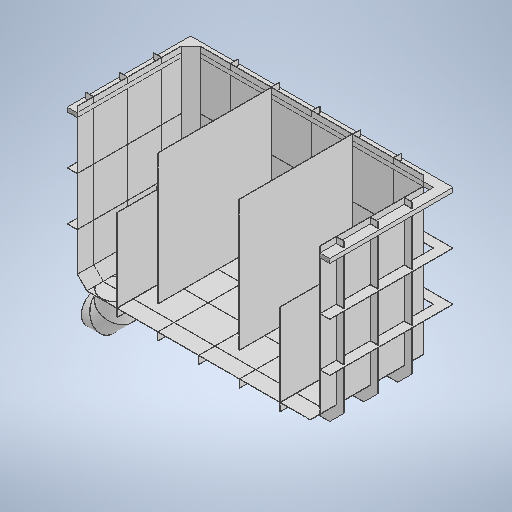
# Autodesk Inventor part: GBK-RK-0003 RK dummy 3
Saved by Autodesk Inventor 2026.2 (Build 302298000, 298)
## iProperties
Created: 2026-08-26
Part Number: GBK-RK-0003 RK dummy 3
Material: Stainless Steel
Document SubType Name: Modeling
Designer: admin
Density: 8 g/cm^3
Appearance: Default
Author: admin
Autodesk Inventor part; units mm, degrees
ref_plane "YZ Plane" through (0, 0, 0) normal (1, 0, 0) x (0, 1, 0)
ref_plane "XZ Plane" through (0, 0, 0) normal (0, 1, 0) x (-1, 0, 0)
ref_plane "XY Plane" through (0, 0, 0) normal (0, 0, 1) x (1, 0, 0)
sketch "Sketch1" plane through (0, 0, 0) normal (0, 1, 0) x (-1, 0, 0)
  line L0 (1250, 650) -> (-1250, 650)
  line L1 (-1250, 650) -> (-1250, -650)
  line L2 (-1250, -650) -> (1250, -650)
  line L3 (1250, -650) -> (1250, 650)
  line L4 (1250, 650) -> (-1250, -650) construction
  line L5 (-1250, 650) -> (1250, -650) construction
  point P0 (0, 0)
  dimension "d0" = 2500
  dimension "d1" = 1300
  constraints: 12 end point, 2 midpoint, 2 parallel, 1 horizontal, 1 perpendicular
  measures "d0" distance of L2.end L1.end
  measures "d1" distance of L1.end L0.end
extrude "Extrusion1" add sketch "Sketch1" along normal blind 100 and the other way blind 1500
chamfer "Chamfer1" distance 100 angle 45 8 edges at (0, -1500, 650) (1250, -1500, 0) (0, -1500, -650) (-1250, -1500, 0) (-1250, -700, 650) (-1250, -700, -650) (1250, -700, -650) (1250, -700, 650)
shell "Shell1" thickness 4 removed faces 1 at (383.3333, 100, -216.6667)
sketch "Sketch4" plane through (0, 0, 0) normal (0, 0, 1) x (1, 0, 0)
  line L0 (-1250, -1400) -> (-1250, 100) projected
  line L1 (-1250, 100) -> (-1250, -1400) projected
  line L2 (-1250, -1400) -> (-1150, -1500) projected
  line L3 (-1150, -1500) -> (-1250, -1400) projected
  line L4 (1150, -1500) -> (-1150, -1500) projected
  line L5 (-1150, -1500) -> (1150, -1500) projected
  line L6 (1250, -1400) -> (1150, -1500) projected
  line L7 (1150, -1500) -> (1250, -1400) projected
  line L8 (1250, 100) -> (1250, -1400) projected
  line L9 (1250, -1400) -> (1250, 100) projected
  line L10 (-1250, 100) -> (-1330, 100)
  line L11 (-1330, 100) -> (-1330, -1433.1371)
  line L12 (-1330, -1433.1371) -> (-1183.1371, -1580)
  line L13 (-1183.1371, -1580) -> (1183.1371, -1580)
  line L14 (1183.1371, -1580) -> (1330, -1433.1371)
  line L15 (1330, -1433.1371) -> (1330, 100)
  line L16 (1330, 100) -> (1250, 100)
  line L17 (0, -1500) -> (0, -1580) construction
  line L18 (-1200, -1450) -> (-1256.5685, -1506.5685) construction
  line L19 (1200, -1450) -> (1256.5685, -1506.5685) construction
  point P0 (0, 0)
  dimension "d16" = 80
  constraints: 20 end point, 7 perpendicular, 6 midpoint, 2 equal length, 2 parallel, 1 point on line
  measures "d16" distance of L1.start L10.end
sketch "Sketch2" plane through (0, 0, 0) normal (1, 0, 0) x (0, 1, 0)
  line L0 (100, -650) -> (100, 650) construction
  line L1 (100, 650) -> (100, 730)
  line L2 (100, 730) -> (-1433.1371, 730)
  line L3 (-1433.1371, 730) -> (-1580, 583.1371)
  line L4 (-1580, 583.1371) -> (-1580, -583.1371)
  line L5 (-1580, -583.1371) -> (-1433.1371, -730)
  line L6 (-1433.1371, -730) -> (100, -730)
  line L7 (100, -730) -> (100, -650)
  line L8 (-1450, -600) -> (-1506.5685, -656.5685) construction
  line L9 (-1500, 0) -> (-1580, 0) construction
  line L10 (-1450, 600) -> (-1506.5685, 656.5685) construction
  line L11 (-1400, -650) -> (-1500, -550)
  line L12 (-1500, -550) -> (-1400, -650) projected
  line L13 (-1400, 650) -> (-1500, 550)
  line L14 (-1500, 550) -> (-1400, 650) projected
  line L15 (-1400, 650) -> (100, 650)
  line L16 (100, 650) -> (-1400, 650) projected
  line L17 (100, -650) -> (-1400, -650)
  line L18 (-1400, -650) -> (100, -650) projected
  line L19 (-1500, -550) -> (-1500, 550) projected
  line L20 (-1500, 550) -> (-1500, -550) projected
  point P0 (0, 0)
  dimension "d10" = 80
  constraints: 30 end point, 6 midpoint, 6 perpendicular, 4 equal length, 2 parallel, 2 point on line
  measures "d10" distance of L0.end L1.end
extrude "Extrusion4" add sketch "Sketch4" along normal mid plane 4
extrude "Extrusion5" add sketch "Sketch2" along normal mid plane 4
pattern_linear "Rectangular Pattern2" count 5 spacing 420 along (1, 0, 0) of "Extrusion5" first direction both ways yes
pattern_linear "Rectangular Pattern3" count 3 spacing 350 along (0, 0, 1) of "Extrusion4" first direction both ways yes
sketch "Sketch5" plane through (0, 0, 0) normal (0, 1, 0) x (-1, 0, 0)
  line L0 (-1246, -548.3431) -> (-1246, 548.3431) projected
  line L1 (-1148.3431, -646) -> (-1246, -548.3431) projected
  line L2 (-1250, -650) -> (1250, -650)
  line L3 (1250, -650) -> (1250, 650)
  line L4 (1250, 650) -> (-1250, 650)
  line L5 (-1250, 650) -> (-1250, -650)
  line L6 (-1250, -650) -> (1250, 650) construction
  line L7 (1250, -650) -> (-1250, 650) construction
  line L8 (1150, 650) -> (842, 650) projected
  line L9 (1250, 352) -> (1250, 550) projected
  line L10 (-1350, -750) -> (1350, -750)
  line L11 (1350, -750) -> (1350, 750)
  line L12 (1350, 750) -> (-1350, 750)
  line L13 (-1350, 750) -> (-1350, -750)
  point P0 (0, 0)
  dimension "d29" = 100
  constraints: 20 end point, 4 parallel, 2 collinear, 2 midpoint, 2 perpendicular, 1 horizontal, 3 other
  measures "d29" distance between parallel lines of L5 L13
extrude "Extrusion6" add sketch "Sketch5" along normal blind 40
extrude "Extrusion7" add sketch "Sketch5" against normal blind 4
pattern_linear "Rectangular Pattern4" count 3 spacing 500 along (0, -1, 0) of "Extrusion7"
sketch "Sketch6" plane through (-838, -4, 730) normal (1, 0, 0) x (0, 0, -1)
  line L0 (84, -1394.3431) -> (84, 104) projected
  line L1 (84, 104) -> (84, -1394.3431) projected
  line L2 (1376, 104) -> (1376, -1394.3431) projected
  line L3 (1376, -1394.3431) -> (1376, 104) projected
  line L4 (1375.6145, -1394.7287) -> (1278.7287, -1491.6145) projected
  line L5 (1375.6145, -1394.7287) -> (1376, -1394.3431) projected
  line L6 (1376, -1394.3431) -> (1375.6145, -1394.7287) projected
  line L7 (1278.7287, -1491.6145) -> (1375.6145, -1394.7287) projected
  line L8 (1278.7287, -1491.6145) -> (1278.3431, -1492) projected
  line L9 (1278.3431, -1492) -> (1278.7287, -1491.6145) projected
  line L10 (1278.3431, -1492) -> (181.6569, -1492) projected
  line L11 (181.6569, -1492) -> (1278.3431, -1492) projected
  line L12 (84.3855, -1394.7287) -> (181.2713, -1491.6145) projected
  line L13 (84.3855, -1394.7287) -> (84, -1394.3431) projected
  line L14 (84, -1394.3431) -> (84.3855, -1394.7287) projected
  line L15 (181.2713, -1491.6145) -> (84.3855, -1394.7287) projected
  line L16 (181.6569, -1492) -> (181.2713, -1491.6145) projected
  line L17 (181.6569, -1492) -> (181.2713, -1491.6145) projected
  line L18 (84, -392) -> (730, -392)
  line L19 (134, -392) -> (194.5, -642)
  line L20 (194.5, -642) -> (619.5, -642)
  line L21 (619.5, -642) -> (680, -392)
  line L22 (730, -392) -> (730, -1492) construction
  line L23 (730, -392) -> (1376, -392)
  line L24 (407, -642) -> (407, -392) construction
  line L25 (1326, -392) -> (1265.5, -642)
  line L26 (1265.5, -642) -> (840.5, -642)
  line L27 (840.5, -642) -> (780, -392)
  point P0 (730, 4)
  point P1 (84, -392)
  point P2 (1376, -1394.3431)
  point P3 (1326, -392)
  dimension "d37" = 425
  dimension "d38" = 1100
  dimension "d39" = 50
  dimension "d40" = 850
  constraints: 20 end point, 4 point on line, 4 symmetric about line, 3 midpoint, 2 perpendicular, 2 vertical, 1 equal length, 1 horizontal, 1 other
  measures "d37" distance of L19.end L20.end
  measures "d38" distance between parallel lines of L10 L18
  measures "d39" distance of L18.start L19.start
  measures "d40" distance between parallel lines of L10 L20
extrude "Extrusion8" add sketch "Sketch6" against normal blind 4 contours L0 L18 L19 L20 L21 L23 L27 L26 L25 L2 L5 L4 L8 L10 L16 L12 L13
mirror "Mirror1" about plane through (0, 0, 0) normal (1, 0, 0) of "Extrusion8"
sketch "Sketch7" plane through (838, -646, 110.5) normal (-1, 0, 0) x (0, 0, 1)
  line L0 (-646, 0) -> (-706.5, 250) projected
  line L1 (-221, 0) -> (-646, 0) projected
  line L2 (-160.5, 250) -> (-221, 0) projected
  line L3 (-706.5, 250) -> (-756.5, 250) projected
  line L4 (-706.5, 250) -> (-160.5, 250)
  point P0 (-110.5, 646)
  constraints: 2 end point, 1 horizontal
extrude "Extrusion9" add sketch "Sketch7" against normal blind 4
sketch "Sketch9" plane through (418, -4, 650) normal (-1, 0, 0) x (0, 0, 1)
  line L0 (-4, -1394.3431) -> (-4, -392) projected
  line L1 (-4, -392) -> (-4, -1394.3431) projected
  line L2 (-4, -1394.3431) -> (-4, -392) projected
  line L3 (-4, -392) -> (-4, -1394.3431) projected
  line L4 (-4, -1394.3431) -> (-4, 104) projected
  line L5 (-4, 104) -> (-4, -1394.3431) projected
  line L6 (-4, -1394.3431) -> (-101.6569, -1492) projected
  line L7 (-101.6569, -1492) -> (-4, -1394.3431) projected
  line L8 (-101.6569, -1492) -> (-1198.3431, -1492) projected
  line L9 (-1198.3431, -1492) -> (-101.6569, -1492) projected
  line L10 (-1198.3431, -1492) -> (-1296, -1394.3431) projected
  line L11 (-1296, -1394.3431) -> (-1198.3431, -1492) projected
  line L12 (-1296, -392) -> (-1296, -1394.3431) projected
  line L13 (-1296, -1394.3431) -> (-1296, 104) projected
  line L14 (-1296, 104) -> (-1296, -1394.3431) projected
  line L15 (-1296, -1394.3431) -> (-1296, -392) projected
  line L16 (-1296, -392) -> (-1296, -1394.3431) projected
  line L17 (-1296, -1394.3431) -> (-1296, -392) projected
  line L18 (0, 104) -> (-100, 104) projected
  line L19 (0, 104) -> (-1296, 104)
  line L20 (0, -1000) -> (0, 44) projected
  line L21 (0, -1242) -> (-1296, -1242)
  point P0 (-650, 4)
  point P1 (0, -1496)
  point P2 (-4, -1242)
  point P3 (-100, 104)
  point P4 (-1296, 104)
  dimension "d65" = 250
  constraints: 4 end point, 2 perpendicular, 2 point on line
  measures "d65" distance between parallel lines of L8 L21
sketch "Sketch10" plane through (-838, -1496, 548.3431) normal (0, 1, 0) x (1, 0, 0)
  line L0 (1676, 0) -> (1676, 1096.6863) projected
  line L1 (1676, 1096.6863) -> (0, 1096.6863) projected
  line L2 (0, 1096.6863) -> (0, 0) projected
  line L3 (0, 0) -> (1676, 0) projected
  circle A0 centre (1476, 350) radius 50
  point P0 (838, 548.3431)
  dimension "d48" = 100
  dimension "d49" = 200
  dimension "d50" = 350
  constraints: 1 centre point
  measures "d48" diameter of A0
  measures "d49" distance from line of A0.centre L0
  measures "d50" distance from line of A0.centre L3
extrude "Extrusion10" add sketch "Sketch10" along normal blind 10 and the other way blind 200 contours A0
sketch "Sketch11" plane through (-1148.3431, 100, -646) normal (0, 0, 1) x (1, 0, 0)
  line L0 (1990.3431, -496) -> (1990.3431, -1498.3431) projected
  line L1 (1990.3431, -1498.3431) -> (2296.6863, -1498.3431) projected
  line L2 (2296.6863, -1498.3431) -> (2296.6863, 0) projected
  line L3 (0, 0) -> (2296.6863, 0) projected
  line L4 (0, 0) -> (0, -1498.3431) projected
  line L5 (0, -1498.3431) -> (306.3431, -1498.3431) projected
  line L6 (306.3431, -1498.3431) -> (306.3431, -496) projected
  line L7 (306.3431, -496) -> (310.3431, -496) projected
  line L8 (310.3431, -496) -> (310.3431, -1498.3431) projected
  line L9 (310.3431, -1498.3431) -> (1986.3431, -1498.3431) projected
  line L10 (1986.3431, -1498.3431) -> (1986.3431, -496) projected
  line L11 (1986.3431, -496) -> (1990.3431, -496) projected
  circle A0 centre (1148.3431, -848.3431) radius 213
  point P0 (1148.3431, -100)
  point P1 (1148.3431, 0)
  dimension "d59" = 426
  dimension "d90" = 650
  constraints: 1 centre point, 1 midpoint, 1 vertical alignment
  measures "d59" diameter of A0
  measures "d90" distance from line of L9 A0.centre
extrude "Extrusion12" add sketch "Sketch11" along normal blind 10 and the other way blind 250 contours A0
extrude "Extrusion13" add sketch "Sketch9" along normal blind 4 contours L21 L12 L13 L19 L18 L4 L0
mirror "Mirror4" about plane through (0, 0, 0) normal (1, 0, 0) of "Extrusion13"
sketch "Sketch12" plane through (-1148.3431, -1496, 548.3431) normal (0, 1, 0) x (1, 0, 0)
  circle A0 centre (136.3431, 200.3431) radius 162.5
  line L0 (-101.6569, 200.3431) -> (-181.6569, 200.3431) projected
  line L1 (-181.6569, 200.3431) -> (-101.6569, 200.3431) projected
  line L2 (306.3431, 12.8431) -> (306.3431, 437.8431) projected
  circle A1 centre (136.3431, 200.3431) radius 159.5
  line L3 (-181.6569, 200.3431) -> (-101.6569, 200.3431) projected
  line L4 (-101.6569, 200.3431) -> (-181.6569, 200.3431) projected
  line L5 (-181.6569, 200.3431) -> (-101.6569, 200.3431) projected
  line L6 (-1.6569, 200.3431) -> (-101.6569, 200.3431) projected
  line L7 (306.3431, 200.3431) -> (-1.6569, 200.3431) projected
  line L8 (306.3431, 200.3431) -> (-34.7939, 200.3431) projected
  line L9 (-34.7939, 200.3431) -> (-181.6569, 200.3431) projected
  line L10 (-101.6569, 200.3431) -> (-181.6569, 200.3431) projected
  line L11 (-181.6569, 200.3431) -> (-101.6569, 200.3431) projected
  point P0 (1148.3431, 548.3431)
  dimension "d68" = 325
  dimension "d71" = 170
  dimension "d72" = 3
  constraints: 2 centre point, 1 point on line
  measures "d68" diameter of A0
  measures "d71" distance from line of A0.centre L2
  measures "d72" radial gap between concentric circles of A0 A1
sketch "Sketch13" plane through (-842, -1580, 348) normal (0, 0, -1) x (-1, 0, 0)
  arc A0 (170, 84) -> (627, -373) centre (627, 84) ccw construction
  line L0 (627, 84) -> (627, -373) construction
  line L1 (627, 84) -> (170, 84) construction
  line L2 (170, 84) -> (170, -68.9332)
  line L3 (0, 80) -> (308, 80) projected
  line L4 (170, -68.9332) -> (274.5574, -173.4907)
  line L5 (274.5574, -173.4907) -> (374.5574, -173.4907)
  line L6 (308, 80) -> (308, 60) construction
  line L7 (341.1371, 0) -> (0, 0) projected
  line L8 (312.2774, -10) -> (27.7226, -127.8665) construction
  line L9 (333.4907, -31.2132) -> (215.6242, -315.7681) construction
  point P0 (-842, 1580)
  dimension "d69" = 90
  dimension "d70" = 457
  dimension "d75" = 135
  dimension "d77" = 20
  dimension "d79" = 100
  dimension "d83" = 10
  dimension "d86" = 45
  dimension "d87" = 67.5
  dimension "d88" = 30
  dimension "d89" = 253.4906
  constraints: 16 end point, 2 equal length, 2 midpoint, 2 perpendicular, 2 point on circle, 1 centre point, 1 horizontal, 1 tangent, 1 vertical
  measures "d69" angle of L1 L0
  measures "d70" radius of A0
  measures "d75" angle of L4 L2
  measures "d77" distance of L3.end L6.end
  measures "d79" distance of L4.end L5.end
  measures "d83" distance from line of L8.start L7
  measures "d86" angle of L8 L9
  measures "d87" angle of L4 L8
  measures "d88" distance of L9.start L8.start
  measures "d89" distance between parallel lines of L5 L3
sweep "Sweep1" add profiles "Sketch12" path "Sketch13" path curves L2 L4 L5 contours L7 A1 L6 A0 | A0 L6 A1 L7
body "Solid1"
